Autodesk Fusion 360 part; units mm, degrees
(part 3 of 3)
  constraint symmetric L502.end L822 L1038.end
  constraint symmetric L503.start L822 L1054.end
  constraint symmetric L504.start L822 L1054.start
  constraint symmetric L506.start L822 L1057.end
  constraint symmetric L506.end L822 L1066.end
  constraint symmetric L507.start L822 L1057.start
  constraint symmetric L508.start L822 L1577.end
  constraint symmetric L510.start L822 L1144.start
  constraint symmetric L510.end L822 L930.start
  constraint symmetric L511.start L822 L913.end
  constraint symmetric L512.start L822 L913.start
  constraint symmetric L514.start L822 L1147.start
  constraint symmetric L514.end L822 L1147.end
  constraint symmetric L515.start L822 L1145.end
  constraint symmetric L516.start L822 L1145.start
  constraint symmetric L518.start L822 L915.start
  constraint symmetric L518.end L822 L915.end
  constraint symmetric L519.start L822 L903.end
  constraint symmetric L520.start L822 L903.start
  constraint symmetric L522.start L822 L1052.end
  constraint symmetric L522.end L822 L1597.start
  constraint symmetric L523.start L822 L1052.start
  constraint symmetric L524.start L822 L1064.start
  constraint symmetric L526.start L822 L1591.start
  constraint symmetric L526.end L822 L1062.start
  constraint symmetric L527.start L822 L1053.end
  constraint symmetric L528.start L822 L1053.start
  constraint symmetric L530.start L822 L1177.start
  constraint symmetric L530.end L822 L1177.end
  constraint symmetric L531.start L822 L928.end
  constraint symmetric L532.start L822 L928.start
  constraint symmetric L534.start L822 L1164.start
  constraint symmetric L534.end L822 L1164.end
  constraint symmetric L535.start L822 L838.end
  constraint symmetric L536.start L822 L838.start
  constraint symmetric L538.start L822 L1072.start
  constraint symmetric L538.end L822 L1072.end
  constraint symmetric L539.start L822 L1163.end
  constraint symmetric L540.start L822 L1079.end
  constraint symmetric L542.start L822 L1223.start
  constraint symmetric L542.end L822 L1223.end
  constraint symmetric L543.start L822 L1083.end
  constraint symmetric L544.start L822 L1083.start
  constraint symmetric L546.start L822 L1225.end
  constraint symmetric L546.end L822 L1047.start
  constraint symmetric L547.start L822 L1225.start
  constraint symmetric L548.start L822 L1047.end
  constraint symmetric L550.start L822 L1340.end
  constraint symmetric L550.end L822 L1494.start
  constraint symmetric L551.start L822 L1340.start
  constraint symmetric L552.start L822 L1434.start
  constraint symmetric L554.start L822 L1344.end
  constraint symmetric L554.end L822 L1480.start
  constraint symmetric L555.start L822 L1343.end
  constraint symmetric L556.start L822 L1343.start
  constraint symmetric L558.start L822 L1316.end
  constraint symmetric L558.end L822 L1324.end
  constraint symmetric L559.start L822 L1316.start
  constraint symmetric L560.start L822 L1332.end
  constraint symmetric L562.start L822 L1368.start
  constraint symmetric L562.end L822 L1319.start
  constraint symmetric L563.start L822 L1320.end
  constraint symmetric L564.start L822 L1319.end
  constraint symmetric L566.start L822 L1443.start
  constraint symmetric L566.end L822 L1443.end
  constraint symmetric L567.start L822 L1496.start
  constraint symmetric L568.start L822 L1505.end
  constraint symmetric L570.start L822 L1435.end
  constraint symmetric L570.end L822 L1436.start
  constraint symmetric L571.start L822 L1345.end
  constraint symmetric L572.start L822 L1345.start
  constraint symmetric L574.start L822 L1352.end
  constraint symmetric L574.end L822 L1328.start
  constraint symmetric L575.start L822 L1299.end
  constraint symmetric L576.start L822 L1299.start
  constraint symmetric L578.start L822 L1354.start
  constraint symmetric L578.end L822 L1346.start
  constraint symmetric L579.start L822 L1504.end
  constraint symmetric L580.start L822 L1346.end
  constraint symmetric L582.start L822 L998.end
  constraint symmetric L582.end L822 L1005.end
  constraint symmetric L583.start L822 L998.start
  constraint symmetric L584.start L822 L999.start
  constraint symmetric L586.start L822 L1171.start
  constraint symmetric L586.end L822 L1021.start
  constraint symmetric L587.start L822 L1172.end
  constraint symmetric L588.start L822 L1021.end
  constraint symmetric L590.start L822 L853.start
  constraint symmetric L590.end L822 L853.end
  constraint symmetric L591.start L822 L845.end
  constraint symmetric L592.start L822 L845.start
  constraint symmetric L594.start L822 L874.start
  constraint symmetric L594.end L822 L872.start
  constraint symmetric L595.start L822 L875.end
  constraint symmetric L596.start L822 L872.end
  constraint symmetric L598.start L822 L1462.start
  constraint symmetric L598.end L822 L1462.end
  constraint symmetric L599.start L822 L1517.end
  constraint symmetric L600.start L822 L1517.start
  constraint symmetric L602.start L822 L1311.start
  constraint symmetric L602.end L822 L1311.end
  constraint symmetric L603.start L822 L1449.end
  constraint symmetric L604.start L822 L1449.start
  constraint symmetric L606.start L822 L1252.end
  constraint symmetric L606.end L822 L1448.end
  constraint symmetric L607.start L822 L1252.start
  constraint symmetric L608.start L822 L1470.end
  constraint symmetric L610.start L822 L1070.end
  constraint symmetric L610.end L822 L1076.start
  constraint symmetric L611.start L822 L1070.start
  constraint symmetric L612.start L822 L1076.end
  constraint symmetric L614.start L822 L1075.start
  constraint symmetric L614.end L822 L1075.end
  constraint symmetric L615.start L822 L1231.end
  constraint symmetric L616.start L822 L1082.end
  constraint symmetric L618.start L822 L1073.start
  constraint symmetric L618.end L822 L1073.end
  constraint symmetric L619.start L822 L1230.start
  constraint symmetric L620.start L822 L1235.end
  constraint symmetric L622.start L822 L1572.end
  constraint symmetric L622.end L822 L1034.start
  constraint symmetric L623.start L822 L1060.end
  constraint symmetric L624.start L822 L1034.end
  constraint symmetric L626.start L822 L1039.start
  constraint symmetric L626.end L822 L1039.end
  constraint symmetric L627.start L822 L1051.end
  constraint symmetric L628.start L822 L1050.end
  constraint symmetric L630.start L822 L917.end
  constraint symmetric L630.end L822 L933.end
  constraint symmetric L631.start L822 L917.start
  constraint symmetric L632.start L822 L924.start
  constraint symmetric L634.start L822 L905.end
  constraint symmetric L634.end L822 L860.start
  constraint symmetric L635.start L822 L905.start
  constraint symmetric L636.start L822 L860.end
  constraint symmetric L638.start L822 L904.end
  constraint symmetric L638.end L822 L847.start
  constraint symmetric L639.start L822 L904.start
  constraint symmetric L640.start L822 L847.end
  constraint symmetric L642.start L822 L1570.end
  constraint symmetric L642.end L822 L1571.start
  constraint symmetric L643.start L822 L1570.start
  constraint symmetric L644.start L822 L1571.end
  constraint symmetric L646.start L822 L1620.end
  constraint symmetric L646.end L822 L1626.end
  constraint symmetric L647.start L822 L1620.start
  constraint symmetric L648.start L822 L1628.start
  constraint symmetric L650.start L822 L911.end
  constraint symmetric L650.end L822 L926.start
  constraint symmetric L651.start L822 L911.start
  constraint symmetric L652.start L822 L926.end
  constraint symmetric L654.start L822 L1160.start
  constraint symmetric L654.end L822 L1160.end
  constraint symmetric L655.start L822 L1143.end
  constraint symmetric L656.start L822 L1143.start
  constraint symmetric L658.start L822 L1077.end
  constraint symmetric L658.end L822 L1215.start
  constraint symmetric L659.start L822 L935.end
  constraint symmetric L660.start L822 L935.start
  constraint symmetric L662.start L822 L1089.start
  constraint symmetric L662.end L822 L1089.end
  constraint symmetric L663.start L822 L1420.end
  constraint symmetric L664.start L822 L1247.end
  constraint symmetric L666.start L822 L1359.start
  constraint symmetric L666.end L822 L1359.end
  constraint symmetric L667.start L822 L1414.end
  constraint symmetric L668.start L822 L1414.start
  constraint symmetric L670.start L822 L1390.start
  constraint symmetric L670.end L822 L1308.start
  constraint symmetric L671.start L822 L1330.end
  constraint symmetric L672.start L822 L1308.end
  constraint symmetric L674.start L822 L1303.start
  constraint symmetric L674.end L822 L1303.end
  constraint symmetric L675.start L822 L1367.start
  constraint symmetric L676.start L822 L1356.end
  constraint symmetric L678.start L822 L1385.start
  constraint symmetric L678.end L822 L1385.end
  constraint symmetric L679.start L822 L1301.end
  constraint symmetric L680.start L822 L1301.start
  constraint symmetric L682.start L822 L1099.start
  constraint symmetric L682.end L822 L1099.end
  constraint symmetric L683.start L822 L1271.start
  constraint symmetric L684.start L822 L1339.end
  constraint symmetric L686.start L822 L1131.end
  constraint symmetric L686.end L822 L1124.start
  constraint symmetric L687.start L822 L1100.end
  constraint symmetric L688.start L822 L1100.start
  constraint symmetric L690.start L822 L1098.end
  constraint symmetric L690.end L822 L1121.start
  constraint symmetric L691.start L822 L1098.start
  constraint symmetric L692.start L822 L1121.end
  constraint symmetric L694.start L822 L1097.end
  constraint symmetric L694.end L822 L1113.end
  constraint symmetric L695.start L822 L1097.start
  constraint symmetric L696.start L822 L1134.start
  constraint symmetric L698.start L822 L1091.end
  constraint symmetric L698.end L822 L1094.start
  constraint symmetric L699.start L822 L1091.start
  constraint symmetric L700.start L822 L1094.end
  constraint symmetric L702.start L822 L1176.end
  constraint symmetric L702.end L822 L1184.end
  constraint symmetric L703.start L822 L1176.start
  constraint symmetric L704.start L822 L1197.end
  constraint symmetric L706.start L822 L1146.start
  constraint symmetric L706.end L822 L1146.end
  constraint symmetric L707.start L822 L1190.start
  constraint symmetric L708.start L822 L1174.end
  constraint symmetric L710.start L822 L848.start
  constraint symmetric L710.end L822 L848.end
  constraint symmetric L711.start L822 L844.end
  constraint symmetric L712.start L822 L844.start
  constraint symmetric L714.start L822 L1554.end
  constraint symmetric L714.end L822 L886.start
  constraint symmetric L715.start L822 L1554.start
  constraint symmetric L716.start L822 L886.end
  constraint symmetric L718.start L822 L1485.end
  constraint symmetric L718.end L822 L1486.end
  constraint symmetric L719.start L822 L1485.start
  constraint symmetric L720.start L822 L1493.start
  constraint symmetric L722.start L822 L1476.end
  constraint symmetric L722.end L822 L1460.start
  constraint symmetric L723.start L822 L1469.end
  constraint symmetric L724.start L822 L1460.end
  constraint symmetric L726.start L822 L1439.start
  constraint symmetric L726.end L822 L1439.end
  constraint symmetric L727.start L822 L1440.start
  constraint symmetric L728.start L822 L1488.end
  constraint symmetric L730.start L822 L1087.end
  constraint symmetric L730.end L822 L1246.end
  constraint symmetric L731.start L822 L1087.start
  constraint symmetric L732.start L822 L1229.start
  constraint symmetric L734.start L822 L1243.end
  constraint symmetric L734.end L822 L1244.start
  constraint symmetric L735.start L822 L1243.start
  constraint symmetric L736.start L822 L1244.end
  constraint symmetric L738.start L822 L1080.start
  constraint symmetric L738.end L822 L1080.end
  constraint symmetric L739.start L822 L1227.end
  constraint symmetric L740.start L822 L1227.start
  constraint symmetric L742.start L822 L1611.start
  constraint symmetric L742.end L822 L1611.end
  constraint symmetric L743.start L822 L1615.end
  constraint symmetric L744.start L822 L1615.start
  constraint symmetric L746.start L822 L1613.end
  constraint symmetric L746.end L822 L1622.end
  constraint symmetric L747.start L822 L1612.end
  constraint symmetric L748.start L822 L1612.start
  constraint symmetric L750.start L822 L836.start
  constraint symmetric L750.end L822 L836.end
  constraint symmetric L751.start L822 L973.start
  constraint symmetric L752.start L822 L953.end
  constraint symmetric L754.start L822 L850.end
  constraint symmetric L754.end L822 L883.end
  constraint symmetric L755.start L822 L850.start
  constraint symmetric L756.start L822 L868.start
  constraint symmetric L758.start L822 L865.start
  constraint symmetric L758.end L822 L865.end
  constraint symmetric L759.start L822 L879.end
  constraint symmetric L760.start L822 L879.start
  constraint symmetric L762.start L822 L1574.end
  constraint symmetric L762.end L822 L1616.end
  constraint symmetric L763.start L822 L1574.start
  constraint symmetric L764.start L822 L1576.start
  constraint symmetric L766.start L822 L1621.end
  constraint symmetric L766.end L822 L1630.start
  constraint symmetric L767.start L822 L1621.start
  constraint symmetric L768.start L822 L1630.end
  constraint symmetric L770.start L822 L942.end
  constraint symmetric L770.end L822 L968.start
  constraint symmetric L771.start L822 L940.end
  constraint symmetric L772.start L822 L940.start
  constraint symmetric L774.start L822 L943.end
  constraint symmetric L774.end L822 L950.start
  constraint symmetric L775.start L822 L943.start
  constraint symmetric L776.start L822 L950.end
  constraint symmetric L778.start L822 L1071.end
  constraint symmetric L778.end L822 L1218.start
  constraint symmetric L779.start L822 L1071.start
  constraint symmetric L780.start L822 L1218.end
  constraint symmetric L782.start L822 L1074.end
  constraint symmetric L782.end L822 L1242.start
  constraint symmetric L783.start L822 L1074.start
  constraint symmetric L784.start L822 L1234.start
  constraint symmetric L786.start L822 L1295.end
  constraint symmetric L786.end L822 L1226.start
  constraint symmetric L787.start L822 L1084.end
  constraint symmetric L788.start L822 L1084.start
  constraint symmetric L790.start L822 L1351.end
  constraint symmetric L790.end L822 L1363.start
  constraint symmetric L791.start L822 L1351.start
  constraint symmetric L792.start L822 L1363.end
  constraint symmetric L794.start L822 L1326.start
  constraint symmetric L794.end L822 L1326.end
  constraint symmetric L795.start L822 L1396.end
  constraint symmetric L796.start L822 L1336.end
  constraint symmetric L798.start L822 L1300.start
  constraint symmetric L798.end L822 L1300.end
  constraint symmetric L799.start L822 L1365.start
  constraint symmetric L800.start L822 L1360.end
  constraint symmetric L802.start L822 L1123.start
  constraint symmetric L802.end L822 L1123.end
  constraint symmetric L803.start L822 L1306.start
  constraint symmetric L804.start L822 L1250.end
  constraint symmetric L806.start L822 L1093.end
  constraint symmetric L806.end L822 L1138.start
  constraint symmetric L807.start L822 L1093.start
  constraint symmetric L808.start L822 L1138.end
  constraint symmetric L810.start L822 L1119.end
  constraint symmetric L810.end L822 L1125.end
  constraint symmetric L811.start L822 L1095.end
  constraint symmetric L812.start L822 L1095.start
  constraint symmetric L814.start L822 L1102.end
  constraint symmetric L814.end L822 L1101.start
  constraint symmetric L815.start L822 L1102.start
  constraint symmetric L816.start L822 L1101.end
  constraint symmetric L818.start L822 L1137.end
  constraint symmetric L818.end L822 L1126.start
  constraint symmetric L819.start L822 L1128.end
  constraint symmetric L820.start L822 L1126.end
  measures "d12" distance of L4.start L6.end
  measures "d14" distance of L11.end L12.end
  measures "d15" distance of L3 P0
  measures "d16" distance of L2 P0
  measures "d23" distance of L10.start L12.end
  measures "d33" distance of L220.start L222.end
  measures "d34" distance of L221.end L222.end
  measures "d35" distance of L6 P5
  measures "d36" distance of L2 P5
extrude "Extrude2" cut sketch "Sketch2" against normal blind 4 contours L0 L2 L4 L5 L6 L7 | L10 L11 L12 L13 | L16 L17 L18 L19 | L20 L21 L22 L23 | L24 L25 L26 L27 | L28 L29 L30 L31 | L32 L33 L34 L35 | L36 L37 L38 L39 | L40 L41 L42 L43 | L44 L45 L46 L47 | L48 L49 L50 L51 | L52 L62 L82 L86 | L53 L56 L59 L69 | L54 L61 L63 L74 | L55 L68 L83 L90 | L57 L64 L71 L89 | L60 L72 L73 L85 | L65 L66 L70 L84 | L67 L87 L91 L92 | L75 L79 L80 L93 | L76 L77 L78 L81 | L94 L104 L124 L128 | L95 L98 L101 L111 | L96 L103 L105 L116 | L97 L110 L125 L132 | L99 L106 L113 L131 | L102 L114 L115 L127 | L107 L108 L112 L126 | L109 L129 L133 L134 | L117 L121 L122 L135 | L118 L119 L120 L123 | L136 L146 L166 L170 | L137 L140 L143 L153 | L138 L145 L147 L158 | L139 L152 L167 L174 | L141 L148 L155 L173 | L144 L156 L157 L169 | L149 L150 L154 L168 | L151 L171 L175 L176 | L159 L163 L164 L177 | L160 L161 L162 L165 | L178 L188 L208 L212 | L179 L182 L185 L195 | L180 L187 L189 L200 | L181 L194 L209 L216 | L183 L190 L197 L215 | L186 L198 L199 L211 | L191 L192 L196 L210 | L193 L213 L217 L218 | L201 L205 L206 L219 | L202 L203 L204 L207 | L220 L221 L222 L223 | L226 L227 L228 L229 | L230 L231 L232 L233 | L234 L235 L236 L237 | L238 L239 L240 L241 | L242 L243 L244 L245 | L246 L247 L248 L249 | L250 L251 L252 L253 | L254 L255 L256 L257 | L258 L259 L260 L261 | L262 L263 L264 L265 | L266 L267 L268 L269 | L270 L271 L272 L273 | L274 L275 L276 L277 | L278 L279 L280 L281 | L282 L283 L284 L285 | L286 L287 L288 L289 | L290 L291 L292 L293 | L294 L295 L296 L297 | L298 L299 L300 L301 | L302 L303 L304 L305 | L306 L307 L308 L309 | L310 L311 L312 L313 | L314 L315 L316 L317 | L318 L319 L320 L321 | L322 L323 L324 L325 | L326 L327 L328 L329 | L330 L331 L332 L333 | L334 L335 L336 L337 | L338 L339 L340 L341 | L342 L343 L344 L345 | L346 L347 L348 L349 | L350 L351 L352 L353 | L354 L355 L356 L357 | L358 L359 L360 L361 | L362 L363 L364 L365 | L366 L367 L368 L369 | L370 L371 L372 L373 | L374 L375 L376 L377 | L378 L379 L380 L381 | L382 L383 L384 L385 | L386 L387 L388 L389 | L390 L391 L392 L393 | L394 L395 L396 L397 | L398 L399 L400 L401 | L402 L403 L404 L405 | L406 L407 L408 L409 | L410 L411 L412 L413 | L414 L415 L416 L417 | L418 L419 L420 L421 | L422 L423 L424 L425 | L426 L427 L428 L429 | L430 L431 L432 L433 | L434 L435 L436 L437 | L438 L439 L440 L441 | L442 L443 L444 L445 | L446 L447 L448 L449 | L450 L451 L452 L453 | L454 L455 L456 L457 | L458 L459 L460 L461 | L462 L463 L464 L465 | L466 L467 L468 L469 | L470 L471 L472 L473 | L474 L475 L476 L477 | L478 L479 L480 L481 | L482 L483 L484 L485 | L486 L487 L488 L489 | L490 L491 L492 L493 | L494 L495 L496 L497 | L498 L499 L500 L501 | L502 L503 L504 L505 | L506 L507 L508 L509 | L510 L511 L512 L513 | L514 L515 L516 L517 | L518 L519 L520 L521 | L522 L523 L524 L525 | L526 L527 L528 L529 | L530 L531 L532 L533 | L534 L535 L536 L537 | L538 L539 L540 L541 | L542 L543 L544 L545 | L546 L547 L548 L549 | L550 L551 L552 L553 | L554 L555 L556 L557 | L558 L559 L560 L561 | L562 L563 L564 L565 | L566 L567 L568 L569 | L570 L571 L572 L573 | L574 L575 L576 L577 | L578 L579 L580 L581 | L582 L583 L584 L585 | L586 L587 L588 L589 | L590 L591 L592 L593 | L594 L595 L596 L597 | L598 L599 L600 L601 | L602 L603 L604 L605 | L606 L607 L608 L609 | L610 L611 L612 L613 | L614 L615 L616 L617 | L618 L619 L620 L621 | L622 L623 L624 L625 | L626 L627 L628 L629 | L630 L631 L632 L633 | L634 L635 L636 L637 | L638 L639 L640 L641 | L642 L643 L644 L645 | L646 L647 L648 L649 | L650 L651 L652 L653 | L654 L655 L656 L657 | L658 L659 L660 L661 | L662 L663 L664 L665 | L666 L667 L668 L669 | L670 L671 L672 L673 | L674 L675 L676 L677 | L678 L679 L680 L681 | L682 L683 L684 L685 | L686 L687 L688 L689 | L690 L691 L692 L693 | L694 L695 L696 L697 | L698 L699 L700 L701 | L702 L703 L704 L705 | L706 L707 L708 L709 | L710 L711 L712 L713 | L714 L715 L716 L717 | L718 L719 L720 L721 | L722 L723 L724 L725 | L726 L727 L728 L729 | L730 L731 L732 L733 | L734 L735 L736 L737 | L738 L739 L740 L741 | L742 L743 L744 L745 | L746 L747 L748 L749 | L750 L751 L752 L753 | L754 L755 L756 L757 | L758 L759 L760 L761 | L762 L763 L764 L765 | L766 L767 L768 L769 | L770 L771 L772 L773 | L774 L775 L776 L777 | L778 L779 L780 L781 | L782 L783 L784 L785 | L786 L787 L788 L789 | L790 L791 L792 L793 | L794 L795 L796 L797 | L798 L799 L800 L801 | L802 L803 L804 L805 | L806 L807 L808 L809 | L810 L811 L812 L813 | L814 L815 L816 L817 | L818 L819 L820 L821 | L823 L1027 L1031 L1206 | L824 L866 L869 L870 | L825 L1041 L1207 L1602 | L826 L900 L1028 L1221 | L827 L829 L831 L833 | L828 L1291 L1415 L1468 | L830 L1023 L1026 L1029 | L832 L897 L901 L1030 | L834 L849 L855 L857 | L835 L837 L843 L871 | L836 L953 L973 L1563 | L838 L1164 L1175 L1178 | L839 L840 L846 L854 | L841 L851 L964 L969 | L842 L861 L956 L1566 | L844 L848 L856 L858 | L845 L853 L859 L862 | L847 L904 L1166 L1185 | L850 L868 L883 L1569 | L852 L873 L945 L1561 | L860 L905 L922 L1149 | L863 L864 L951 L955 | L865 L879 L941 L957 | L867 L948 L1025 L1568 | L872 L874 L875 L884 | L876 L877 L966 L971 | L880 L881 L882 L885 | L886 L1554 L1555 L1559 | L887 L944 L970 L1564 | L888 L889 L954 L965 | L890 L899 L1423 L1625 | L891 L939 L967 L972 | L892 L947 L952 L1024 | L893 L1048 L1219 L1220 | L894 L895 L898 L1222 | L896 L1081 L1276 L1477 | L902 L1205 L1208 L1209 | L903 L915 L1151 L1159 | L906 L975 L1007 L1020 | L907 L909 L923 L925 | L908 L912 L929 L1139 | L910 L1152 L1167 L1203 | L911 L926 L1142 L1183 | L913 L930 L1144 L1148 | L914 L916 L921 L997 | L917 L924 L933 L1157 | L918 L920 L931 L936 | L919 L934 L1153 L1182 | L927 L1019 L1170 L1189 | L928 L1177 L1188 L1192 | L935 L1077 L1215 L1416 | L937 L1140 L1162 L1168 | L940 L942 L968 L1558 | L943 L950 L1560 L1562 | L946 L1553 L1557 L1565 | L949 L958 L961 L963 | L960 L1037 L1042 L1607 | L962 L984 L1043 L1044 | L974 L1003 L1017 L1181 | L976 L979 L985 L987 | L977 L986 L996 L1010 | L978 L980 L981 L1608 | L982 L1008 L1009 L1158 | L983 L1016 L1022 L1191 | L988 L1603 L1604 L1606 | L989 L1011 L1013 L1018 | L990 L993 L1006 L1196 | L991 L994 L1001 L1012 | L992 L995 L1000 L1015 | L998 L999 L1005 L1014 | L1002 L1212 L1217 L1224 | L1004 L1069 L1211 L1216 | L1021 L1171 L1172 L1193 | L1032 L1033 L1575 L1596 | L1034 L1060 L1572 L1578 | L1035 L1063 L1589 L1595 | L1036 L1049 L1590 L1592 | L1038 L1054 L1058 L1593 | L1039 L1050 L1051 L1580 | L1040 L1573 L1583 L1584 | L1045 L1059 L1585 L1587 | L1046 L1061 L1067 L1600 | L1047 L1225 L1428 L1542 | L1052 L1064 L1597 L1598 | L1053 L1062 L1591 L1594 | L1055 L1068 L1581 L1588 | L1056 L1065 L1582 L1586 | L1057 L1066 L1577 L1599 | L1070 L1076 L1236 L1432 | L1071 L1218 L1425 L1567 | L1072 L1079 L1163 L1210 | L1073 L1230 L1235 L1241 | L1074 L1234 L1242 L1419 | L1075 L1082 L1231 L1430 | L1078 L1232 L1418 L1453 | L1080 L1227 L1228 L1429 | L1083 L1223 L1237 L1238 | L1084 L1226 L1295 L1335 | L1085 L1088 L1240 L1422 | L1086 L1266 L1288 L1534 | L1087 L1229 L1246 L1427 | L1089 L1247 L1420 L1424 | L1090 L1371 L1397 L1402 | L1091 L1094 L1110 L1129 | L1092 L1130 L1378 L1380 | L1093 L1138 L1383 L1411 | L1095 L1119 L1125 L1362 | L1096 L1347 L1394 L1398 | L1097 L1113 L1134 L1412 | L1098 L1121 L1333 L1393 | L1099 L1271 L1339 L1374 | L1100 L1124 L1131 L1358 | L1101 L1102 L1103 L1117 | L1104 L1106 L1135 L1387 | L1105 L1369 L1401 L1409 | L1107 L1136 L1366 L1391 | L1108 L1114 L1118 L1379 | L1109 L1122 L1132 L1377 | L1111 L1313 L1375 L1399 | L1112 L1361 L1386 L1405 | L1115 L1120 L1408 L1413 | L1116 L1127 L1133 L1384 | L1123 L1250 L1306 L1325 | L1126 L1128 L1137 L1364 | L1141 L1150 L1156 L1161 | L1143 L1160 L1179 L1198 | L1145 L1147 L1154 L1200 | L1146 L1174 L1190 L1199 | L1165 L1186 L1201 L1204 | L1173 L1180 L1194 L1195 | L1176 L1184 L1197 L1202 | L1213 L1265 L1274 L1283 | L1214 L1253 L1286 L1433 | L1233 L1239 L1245 L1417 | L1243 L1244 L1248 L1426 | L1249 L1444 L1459 L1489 | L1251 L1259 L1446 L1487 | L1252 L1448 L1470 L1511 | L1254 L1287 L1289 L1458 | L1255 L1279 L1463 L1481 | L1257 L1268 L1275 L1277 | L1258 L1260 L1452 L1479 | L1261 L1296 L1442 L1475 | L1262 L1278 L1293 L1294 | L1263 L1282 L1467 L1471 | L1267 L1270 L1273 L1285 | L1269 L1280 L1297 L1490 | L1272 L1281 L1292 L1474 | L1290 L1451 L1465 L1472 | L1298 L1307 L1331 L1513 | L1299 L1328 L1352 L1495 | L1300 L1360 L1365 L1400 | L1301 L1385 L1388 L1406 | L1302 L1329 L1509 L1515 | L1303 L1356 L1367 L1376 | L1304 L1342 L1350 L1454 | L1305 L1317 L1355 L1521 | L1308 L1330 L1390 L1546 | L1309 L1321 L1382 L1524 | L1310 L1334 L1357 L1545 | L1311 L1449 L1506 L1536 | L1312 L1466 L1537 L1552 | L1314 L1491 L1550 L1551 | L1315 L1322 L1450 L1507 | L1316 L1324 L1332 L1337 | L1318 L1497 L1501 L1508 | L1319 L1320 L1368 L1532 | L1323 L1437 L1461 L1464 | L1326 L1336 L1396 L1548 | L1327 L1373 L1389 L1404 | L1338 L1499 L1533 L1547 | L1340 L1434 L1494 L1526 | L1341 L1348 L1392 L1543 | L1343 L1344 L1480 L1527 | L1345 L1435 L1436 L1516 | L1346 L1354 L1504 L1518 | L1349 L1457 L1482 L1503 | L1351 L1363 L1407 L1525 | L1353 L1512 L1531 L1544 | L1359 L1414 L1421 L1431 | L1370 L1395 L1510 L1540 | L1372 L1381 L1403 L1410 | L1438 L1478 L1530 L1538 | L1439 L1440 L1488 L1549 | L1443 L1496 L1505 L1539 | L1445 L1455 L1484 L1522 | L1447 L1492 L1502 L1514 | L1456 L1520 L1529 L1535 | L1460 L1469 L1476 L1541 | L1462 L1517 L1523 L1528 | L1473 L1483 L1500 L1519 | L1485 L1486 L1493 L1498 | L1570 L1571 L1579 L1634 | L1574 L1576 L1616 L1618 | L1601 L1605 L1610 L1623 | L1609 L1614 L1619 L1627 | L1611 L1615 L1617 L1629 | L1612 L1613 L1622 L1624 | L1620 L1626 L1628 L1633 | L1621 L1630 L1631 L1632
extrude "Extrude3" add sketch "Sketch1" along normal blind 6 contours L3 A4 | L2 A0 | L3 A2 | L2 A1 | L3 A3 picked at (42.013, 22.1964) picked at (-26.7233, -27.0112) picked at (41.5189, -0.097) picked at (27.2908, -26.9155) picked at (41.4524, -22.1764)
equation "bb_length = 82 mm"
equation "bb_width = 53 mm"
equation "bb_height = 10 mm"
equation "valley_width = 2 mm"
equation "pin_spacing = 1.25 mm"
equation "pin_spacing_real = 2.5 mm"
equation "d27 = -pin_spacing_real * 4"
equation "d40 = pin_spacing_real * 4"

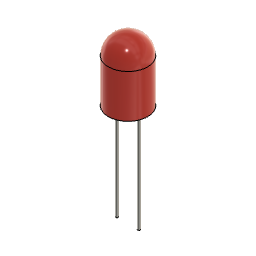
design "LED"
Autodesk Fusion 360 part; units mm, degrees
sketch "Sketch2" plane through (0, 0, 0) normal (1, 0, 0) x (0, 1, 0)
  line L0 (2.5, 0) -> (2.5, 5.5)
  line L1 (2.5, 0) -> (0, 0)
  line L2 (-0.25, 0) -> (0, 0)
  line L3 (0, 0) -> (0, 10.8264)
  circle A0 centre (0, 5.5) radius 2.5
  line L4 (0, 0) -> (0, 3)
  dimension "d1" = 5.5
  dimension "d2" = 2.5
  constraint vertical L0
  constraint coincident L1.end L2.end
  constraint perpendicular L1 L3
  constraint coincident L3 A0.centre
  constraint coincident L0.end A0
  constraint coincident A0 L4.end
  constraint coincident L3 L4.end
  constraint perpendicular L2 L4
  measures "d1" distance of L0.start L0.end
  measures "d2" distance of L1.end L0.start
revolve "Revolve2" add sketch "Sketch2" angle 360 about axis through (0, 0, 0) along (0, 0, 1) contours L0 L1 L3 A0 L4 | L3 A0 picked at (0.7484, 6.0542)
sketch "Sketch4" plane through (0, 0, 0) normal (0, 0, -1) x (1, 0, 0)
  circle A0 centre (0, 0) radius 2.5
  line L0 (0, 0) -> (-2.5, 0) construction
  circle A1 centre (-1.4, 0) radius 0.15
  line L1 (0, 0.25) -> (0, 0)
  circle A2 centre (1.4, 0) radius 0.15
  dimension "d8" = 0.3
  constraint coincident A0.centre L0.start
  constraint coincident A0 L0.end
  constraint horizontal L0
  constraint coincident L0 A1.centre
  constraint symmetric A1 L1 A2
  measures "d8" diameter of A1
extrude "Extrude2" add sketch "Sketch4" along normal blind 13 contours A1 | A2
equation "d2 = 0.5 cm / 2"

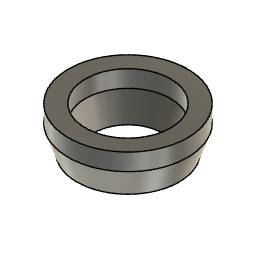
design "Button Housing"
Autodesk Fusion 360 part; units mm, degrees
sketch "Sketch1" plane through (0, 0, 0) normal (0, 1, 0) x (1, 0, 0)
  line L0 (4, -8.2169) -> (5, -11.2169)
  line L1 (5, -11.2169) -> (7, -11.2169)
  line L2 (7, -11.2169) -> (6, -8.2169)
  line L3 (6, -8.2169) -> (4, -8.2169)
  line L4 (-22, 0) -> (16.2899, 0) construction
  line L5 (5, -11.2169) -> (7, -11.2169)
  line L6 (7, -11.2169) -> (7, -13.2169)
  line L7 (7, -13.2169) -> (5, -13.2169)
  line L8 (5, -13.2169) -> (5, -11.2169)
  line L9 (0, -21) -> (0, 5.3257) construction
  dimension "d1" = 2
  dimension "d2" = 2
  dimension "d3" = 3
  dimension "d4" = 2
  dimension "d5" = 4
  dimension "d6" = 1
  constraint horizontal L1
  constraint parallel L0 L2
  constraint horizontal L4
  constraint parallel L3 L4
  constraint horizontal L5
  constraint vertical L6
  constraint horizontal L7
  constraint vertical L8
  constraint perpendicular L4 L9
  measures "d1" distance of L0.start L2.end
  measures "d2" distance of L1.end L6.end
  measures "d3" distance of L3 L5
  measures "d4" distance of L6.end L7.end
  measures "d5" distance of L0.start L9
  measures "d6" distance of L0.start L8
revolve "Revolve1" add sketch "Sketch1" angle 360 about axis through (0, 0, 21) along (0, 0, -1)

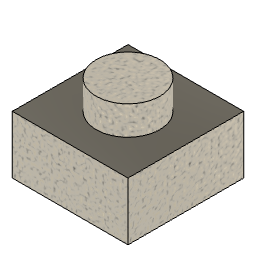
design "Button"
Autodesk Fusion 360 part; units mm, degrees
sketch "Sketch1" plane through (0, 0, 0) normal (0, 0, 1) x (1, 0, 0)
  line L0 (0, 0) -> (6, 0)
  line L1 (6, 0) -> (6, 6)
  line L2 (6, 6) -> (0, 6)
  line L3 (0, 6) -> (0, 0)
  dimension "d1" = 6
  dimension "d2" = 6
  constraint horizontal L0
  constraint vertical L1
  constraint horizontal L2
  constraint vertical L3
  constraint coincident L0.start L3.end
  measures "d1" distance of L0.start L0.end
  measures "d2" distance of L0.start L2.end
extrude "Extrude1" add sketch "Sketch1" along normal blind 3
sketch "Sketch2" plane through (0, 0, 3) normal (0, 0, 1) x (-1, 0, 0)
  line L0 (0, -6) -> (0, 0)
  line L1 (0, 0) -> (-6, 0)
  line L2 (-6, 0) -> (-6, -6)
  line L3 (-6, -6) -> (0, -6)
  circle A0 centre (-3, -3) radius 1.65
  line L4 (-3, 0) -> (-3, -6) construction
  line L5 (0, -3) -> (-6, -3) construction
  dimension "d5" = 3.3
  constraint midpoint L1 L4.start
  constraint midpoint L3 L4.end
  constraint midpoint L0 L5.start
  constraint midpoint L2 L5.end
  measures "d5" diameter of A0
extrude "Extrude2" add sketch "Sketch2" along normal blind 1.5 contours A0
